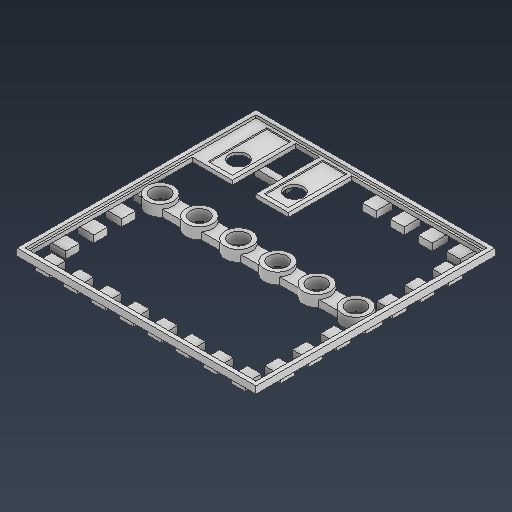
# Autodesk Inventor part: Faceplate
Saved by Autodesk Inventor 2025.3 (Build 293356000, 356)
## iProperties
Created: 2025-09-08
Part Number: Faceplate
Material: Generic
Document SubType Name: Modeling
Designer: tolga
Density: 1 g/cm^3
Appearance: Default
Author: tolga
Autodesk Inventor part; units mm, degrees
ref_plane "YZ Plane" through (0, 0, 0) normal (1, 0, 0) x (0, 1, 0)
ref_plane "XZ Plane" through (0, 0, 0) normal (0, 1, 0) x (-1, 0, 0)
ref_plane "XY Plane" through (0, 0, 0) normal (0, 0, 1) x (1, 0, 0)
sketch "Sketch1" plane through (0, 0, 0) normal (0, 1, 0) x (-1, 0, 0)
  line L0 (0, 0) -> (-171, 0)
  line L1 (-171, 0) -> (-171, -171)
  line L2 (-171, -171) -> (0, -171)
  line L3 (0, -171) -> (0, 0)
  dimension "d0" = 171
  dimension "d1" = 171
  constraints: 8 end point, 2 parallel, 1 horizontal, 1 perpendicular
  measures "d0" distance of L2.end L1.end
  measures "d1" distance of L1.end L0.end
extrude "Extrusion1" add sketch "Sketch1" along normal blind 3
sketch "Sketch3" plane through (0, 3, 0) normal (0, 1, 0) x (1, 0, 0)
  line L0 (4, 64) -> (82, 64) construction
  line L1 (82, 64) -> (82, 4) construction
  line L2 (82, 4) -> (4, 4) construction
  line L3 (4, 4) -> (4, 64) construction
  line L4 (89, 107) -> (167, 107) construction
  line L5 (167, 107) -> (167, 167) construction
  line L6 (167, 167) -> (89, 167) construction
  line L7 (89, 167) -> (89, 107) construction
  line L8 (4, 167) -> (79, 167) construction
  line L9 (79, 167) -> (79, 102) construction
  line L10 (4, 72) -> (4, 167) construction
  line L11 (4, 72) -> (167, 72) construction
  line L12 (167, 72) -> (167, 102) construction
  line L13 (167, 102) -> (79, 102) construction
  line L14 (87, 67) -> (167, 67) construction
  line L15 (167, 67) -> (167, 37) construction
  line L16 (167, 37) -> (87, 37) construction
  line L17 (87, 37) -> (87, 67) construction
  line L18 (87, 32) -> (167, 32) construction
  line L19 (167, 32) -> (167, 7) construction
  line L20 (167, 7) -> (87, 7) construction
  line L21 (87, 7) -> (87, 32) construction
  line L22 (10.3, 32) -> (25.7, 32)
  line L23 (25.7, 32) -> (25.7, 16.6)
  line L24 (25.7, 16.6) -> (10.3, 16.6)
  line L25 (10.3, 16.6) -> (10.3, 32)
  line L26 (10.3, 60) -> (25.7, 60)
  line L27 (10.3, 44.6) -> (10.3, 60)
  line L28 (25.7, 44.6) -> (10.3, 44.6)
  line L29 (25.7, 60) -> (25.7, 44.6)
  line L30 (35.3, 32) -> (50.7, 32)
  line L31 (35.3, 16.6) -> (35.3, 32)
  line L32 (50.7, 16.6) -> (35.3, 16.6)
  line L33 (50.7, 32) -> (50.7, 16.6)
  line L34 (35.3, 60) -> (50.7, 60)
  line L35 (35.3, 44.6) -> (35.3, 60)
  line L36 (50.7, 44.6) -> (35.3, 44.6)
  line L37 (50.7, 60) -> (50.7, 44.6)
  line L38 (60.3, 32) -> (75.7, 32)
  line L39 (60.3, 16.6) -> (60.3, 32)
  line L40 (75.7, 16.6) -> (60.3, 16.6)
  line L41 (75.7, 32) -> (75.7, 16.6)
  line L42 (60.3, 60) -> (75.7, 60)
  line L43 (60.3, 44.6) -> (60.3, 60)
  line L44 (75.7, 44.6) -> (60.3, 44.6)
  line L45 (75.7, 60) -> (75.7, 44.6)
  line L46 (10.3, 60) -> (10.3, 16.6) construction
  line L47 (10.3, 60) -> (75.7, 60) construction
  line L48 (95.3, 135) -> (110.7, 135)
  line L49 (110.7, 135) -> (110.7, 119.6)
  line L50 (110.7, 119.6) -> (95.3, 119.6)
  line L51 (95.3, 119.6) -> (95.3, 135)
  line L52 (95.3, 163) -> (110.7, 163)
  line L53 (95.3, 147.6) -> (95.3, 163)
  line L54 (110.7, 147.6) -> (95.3, 147.6)
  line L55 (110.7, 163) -> (110.7, 147.6)
  line L56 (120.3, 135) -> (135.7, 135)
  line L57 (120.3, 119.6) -> (120.3, 135)
  line L58 (135.7, 119.6) -> (120.3, 119.6)
  line L59 (135.7, 135) -> (135.7, 119.6)
  line L60 (120.3, 163) -> (135.7, 163)
  line L61 (120.3, 147.6) -> (120.3, 163)
  line L62 (135.7, 147.6) -> (120.3, 147.6)
  line L63 (135.7, 163) -> (135.7, 147.6)
  line L64 (145.3, 135) -> (160.7, 135)
  line L65 (145.3, 119.6) -> (145.3, 135)
  line L66 (160.7, 119.6) -> (145.3, 119.6)
  line L67 (160.7, 135) -> (160.7, 119.6)
  line L68 (145.3, 163) -> (160.7, 163)
  line L69 (145.3, 147.6) -> (145.3, 163)
  line L70 (160.7, 147.6) -> (145.3, 147.6)
  line L71 (160.7, 163) -> (160.7, 147.6)
  line L72 (95.3, 163) -> (95.3, 119.6) construction
  line L73 (95.3, 163) -> (160.7, 163) construction
  circle A0 centre (107, 52) radius 12.5 construction
  circle A1 centre (147, 52) radius 12.5 construction
  circle A2 centre (107, 52) radius 4
  circle A3 centre (147, 52) radius 4
  circle A4 centre (99, 19.5) radius 8.1 construction
  circle A5 centre (127, 19.5) radius 8.1 construction
  circle A6 centre (155, 19.5) radius 8.1 construction
  circle A7 centre (99, 19.5) radius 6.4
  circle A8 centre (127, 19.5) radius 6.4
  circle A9 centre (155, 19.5) radius 6.4
  circle A10 centre (155.5, 87) radius 6.5
  circle A11 centre (127.5, 87) radius 6.5
  circle A12 centre (99.5, 87) radius 6.5
  circle A13 centre (71.5, 87) radius 6.5
  circle A14 centre (43.5, 87) radius 6.5
  circle A15 centre (15.5, 87) radius 6.5
  circle A16 centre (61.5, 137) radius 6.5
  circle A17 centre (21.5, 137) radius 6.5
  line L74 (0, 171) -> (0, 0) projected
  line L75 (171, 171) -> (0, 171) projected
  line L76 (171, 0) -> (171, 171) projected
  line L77 (0, 0) -> (171, 0) projected
  point P0 (4, 34)
  point P1 (43, 60)
  point P2 (43, 64)
  point P3 (18, 44.6)
  point P4 (25.7, 52.3)
  point P5 (128, 163)
  point P6 (103, 147.6)
  point P7 (110.7, 155.3)
  point P8 (128, 163)
  point P9 (128, 107)
  point P10 (87, 52)
  point P11 (167, 19.5)
  point P12 (167, 87)
  point P13 (79, 134.5)
  dimension "d9" = 60
  dimension "d10" = 78
  dimension "d11" = 78
  dimension "d12" = 60
  dimension "d17" = 75
  dimension "d20" = 5
  dimension "d21" = 30
  dimension "d22" = 5
  dimension "d23" = 5
  dimension "d27" = 5
  dimension "d28" = 5
  dimension "d31" = 25
  dimension "d32" = 15.4
  dimension "d33" = 15.4
  dimension "d37" = 28
  dimension "d40" = 25
  dimension "d43" = 12.6
  dimension "d44" = 6.3
  dimension "d45" = 4
  dimension "d46" = 14
  dimension "d47" = 11.7
  dimension "d52" = 15.4
  dimension "d53" = 15.4
  dimension "d54" = 28
  dimension "d55" = 25
  dimension "d56" = 12.6
  dimension "d57" = 30
  dimension "d58" = 80
  dimension "d59" = 25
  dimension "d60" = 25
  dimension "d61" = 20
  dimension "d62" = 40
  dimension "d63" = 8
  dimension "d64" = 8
  dimension "d67" = 80
  dimension "d68" = 16.2
  dimension "d69" = 16.2
  dimension "d70" = 16.2
  dimension "d71" = 28
  dimension "d72" = 28
  dimension "d73" = 12
  dimension "d74" = 12.8
  dimension "d75" = 12.8
  dimension "d76" = 12.8
  dimension "d77" = 13
  dimension "d80" = 28
  dimension "d85" = 11.5
  dimension "d86" = 163
  dimension "d87" = 65
  dimension "d88" = 95
  dimension "d89" = 88
  dimension "d90" = 13
  dimension "d91" = 13
  dimension "d92" = 30
  dimension "d93" = 40
  dimension "d94" = 17.5
  dimension "d105" = 4
  dimension "d106" = 4
  dimension "d107" = 4
  dimension "d108" = 4
  dimension "d109" = 4
  dimension "d110" = 4
  dimension "d111" = 7
  dimension "d112" = 4
  constraints: 148 end point, 18 centre point, 14 midpoint, 13 parallel, 11 horizontal, 11 perpendicular, 7 horizontal alignment, 6 collinear, 5 coincident, 2 vertical, 2 vertical alignment, 86 other
  measures "d9" distance between parallel lines of L2 L0
  measures "d10" distance between parallel lines of L3 L1
  measures "d11" distance of L6.end L5.end
  measures "d12" distance of L5.end L4.end
  measures "d17" distance between parallel lines of L10 L9
  measures "d20" distance between parallel lines of L4 L13
  measures "d21" distance between parallel lines of L13 L11
  measures "d22" distance between parallel lines of L11 L14
  measures "d23" distance between parallel lines of L1 L17
  measures "d27" distance between parallel lines of L1 L21
  measures "d28" distance between parallel lines of L16 L18
  measures "d31" distance between parallel lines of L20 L18
  measures "d32" distance of L23.end L24.end
  measures "d33" distance of L22.end L23.end
  measures "d37" distance of L23.end L28.start
  measures "d40" distance of L23.end L32.start
  measures "d43" distance between parallel lines of L2 L24
  measures "d44" distance between parallel lines of L3 L27
  measures "d45" distance between parallel lines of L0 L47
  measures "d46" distance from line of L3 point (18, 44.6)
  measures "d47" distance from line of L0 point (25.7, 52.3)
  measures "d52" distance of L49.end L72.end
  measures "d53" distance of L49.start L49.end
  measures "d54" distance of L49.end L54.start
  measures "d55" distance of L49.end L58.start
  measures "d56" distance between parallel lines of L4 L50
  measures "d57" distance between parallel lines of L14 L16
  measures "d58" distance between parallel lines of L15 L17
  measures "d59" diameter of A0
  measures "d60" diameter of A1
  measures "d61" distance from line of L17 A0.centre
  measures "d62" distance of A0.centre A1.centre
  measures "d63" diameter of A2
  measures "d64" diameter of A3
  measures "d67" distance between parallel lines of L19 L21
  measures "d68" diameter of A4
  measures "d69" diameter of A5
  measures "d70" diameter of A6
  measures "d71" distance of A5.centre A4.centre
  measures "d72" distance of A6.centre A5.centre
  measures "d73" distance from line of L21 A4.centre
  measures "d74" diameter of A7
  measures "d75" diameter of A8
  measures "d76" diameter of A9
  measures "d77" diameter of A10
  measures "d80" distance of A10.centre A11.centre
  measures "d85" distance from line of L12 A10.centre
  measures "d86" distance of L10.start L11.end
  measures "d87" distance of L8.end L9.end
  measures "d88" distance of L10.start L8.start
  measures "d89" distance of L12.end L9.end
  measures "d90" diameter of A16
  measures "d91" diameter of A17
  measures "d92" distance from line of L8 A17.centre
  measures "d93" distance of A17.centre A16.centre
  measures "d94" horizontal distance of point (79, 134.5) A16.centre
  measures "d105" distance between parallel lines of L74 L10
  measures "d106" distance between parallel lines of L75 L8
  measures "d107" distance between parallel lines of L75 L6
  measures "d108" distance between parallel lines of L76 L5
  measures "d109" distance between parallel lines of L76 L12
  measures "d110" distance between parallel lines of L76 L15
  measures "d111" distance between parallel lines of L77 L20
  measures "d112" distance between parallel lines of L76 L19
extrude "Extrusion3" cut sketch "Sketch3" against normal up to surface (3 mm away) contours L22 L23 L24 L25 | L26 L29 L28 L27 | L30 L33 L32 L31 | L34 L37 L36 L35 | L38 L41 L40 L39 | L42 L45 L44 L43 | L48 L49 L50 L51 | L52 L55 L54 L53 | L56 L59 L58 L57 | L60 L63 L62 L61 | L64 L67 L66 L65 | L68 L71 L70 L69 | A2 | A3 | A7 | A8 | A9 | A10 | A11 | A12 | A13 | A14 | A15 | A16 | A17
sketch "Sketch5" plane through (0, 3, 0) normal (0, 1, 0) x (1, 0, 0)
  circle A0 centre (21.5, 137) radius 6.5 construction
  circle A1 centre (61.5, 137) radius 6.5 construction
  line L0 (12.9, 165.8) -> (30.1, 165.8)
  line L1 (30.1, 165.8) -> (30.1, 124)
  line L2 (30.1, 124) -> (12.9, 124)
  line L3 (12.9, 124) -> (12.9, 165.8)
  line L4 (70.1, 124) -> (52.9, 124)
  line L5 (52.9, 124) -> (52.9, 165.8)
  line L6 (52.9, 165.8) -> (70.1, 165.8)
  line L7 (70.1, 165.8) -> (70.1, 124)
  point P0 (0, 0)
  point P1 (21.5, 165.8)
  point P2 (61.5, 165.8)
  point P3 (61.5, 124)
  point P4 (21.5, 124)
  dimension "d99" = 13
  dimension "d100" = 28.8
  dimension "d101" = 17.2
  dimension "d102" = 17.2
  constraints: 16 end point, 4 midpoint, 4 parallel, 2 horizontal, 2 horizontal alignment, 2 perpendicular, 2 vertical alignment
  measures "d99" distance from line of L2 A0.centre
  measures "d100" distance of point (21.5, 165.8) A0.centre
  measures "d101" distance between parallel lines of L1 L3
  measures "d102" distance between parallel lines of L7 L5
extrude "Extrusion5" cut sketch "Sketch5" against normal blind 1
sketch "Sketch7" plane through (0, 3, 0) normal (0, 1, 0) x (1, 0, 0)
  line L0 (52.9, 124) -> (52.9, 165.8) projected
  line L1 (52.9, 165.8) -> (70.1, 165.8) projected
  line L2 (70.1, 165.8) -> (70.1, 124) projected
  line L3 (70.1, 124) -> (52.9, 124) projected
  line L4 (30.1, 165.8) -> (30.1, 124) projected
  line L5 (30.1, 124) -> (12.9, 124) projected
  line L6 (12.9, 124) -> (12.9, 165.8) projected
  line L7 (12.9, 165.8) -> (30.1, 165.8) projected
  circle A0 centre (15.5, 87) radius 6.5 projected
  circle A1 centre (71.5, 87) radius 6.5 projected
  circle A2 centre (99, 19.5) radius 6.4 projected
  line L8 (35.3, 44.6) -> (35.3, 60) projected
  line L9 (35.3, 60) -> (50.7, 60) projected
  line L10 (50.7, 60) -> (50.7, 44.6) projected
  line L11 (50.7, 44.6) -> (35.3, 44.6) projected
  line L12 (50.7, 16.6) -> (35.3, 16.6) projected
  line L13 (35.3, 16.6) -> (35.3, 32) projected
  line L14 (35.3, 32) -> (50.7, 32) projected
  line L15 (50.7, 32) -> (50.7, 16.6) projected
  line L16 (120.3, 119.6) -> (120.3, 135) projected
  line L17 (120.3, 135) -> (135.7, 135) projected
  line L18 (135.7, 135) -> (135.7, 119.6) projected
  line L19 (135.7, 119.6) -> (120.3, 119.6) projected
  circle A3 centre (107, 52) radius 4 projected
  line L20 (145.3, 163) -> (160.7, 163) projected
  line L21 (160.7, 163) -> (160.7, 147.6) projected
  line L22 (160.7, 147.6) -> (145.3, 147.6) projected
  line L23 (145.3, 147.6) -> (145.3, 163) projected
  line L24 (110.7, 135) -> (110.7, 119.6) projected
  line L25 (110.7, 119.6) -> (95.3, 119.6) projected
  line L26 (95.3, 119.6) -> (95.3, 135) projected
  line L27 (95.3, 135) -> (110.7, 135) projected
  line L28 (60.3, 44.6) -> (60.3, 60) projected
  line L29 (60.3, 60) -> (75.7, 60) projected
  line L30 (75.7, 60) -> (75.7, 44.6) projected
  line L31 (75.7, 44.6) -> (60.3, 44.6) projected
  circle A4 centre (127, 19.5) radius 6.4 projected
  circle A5 centre (99.5, 87) radius 6.5 projected
  circle A6 centre (43.5, 87) radius 6.5 projected
  circle A7 centre (155.5, 87) radius 6.5 projected
  line L32 (10.3, 44.6) -> (10.3, 60) projected
  line L33 (10.3, 60) -> (25.7, 60) projected
  line L34 (25.7, 60) -> (25.7, 44.6) projected
  line L35 (25.7, 44.6) -> (10.3, 44.6) projected
  line L36 (25.7, 16.6) -> (10.3, 16.6) projected
  line L37 (10.3, 16.6) -> (10.3, 32) projected
  line L38 (10.3, 32) -> (25.7, 32) projected
  line L39 (25.7, 32) -> (25.7, 16.6) projected
  line L40 (120.3, 147.6) -> (120.3, 163) projected
  line L41 (120.3, 163) -> (135.7, 163) projected
  line L42 (135.7, 163) -> (135.7, 147.6) projected
  line L43 (135.7, 147.6) -> (120.3, 147.6) projected
  circle A8 centre (147, 52) radius 4 projected
  line L44 (145.3, 135) -> (160.7, 135) projected
  line L45 (160.7, 135) -> (160.7, 119.6) projected
  line L46 (160.7, 119.6) -> (145.3, 119.6) projected
  line L47 (145.3, 119.6) -> (145.3, 135) projected
  line L48 (110.7, 147.6) -> (95.3, 147.6) projected
  line L49 (95.3, 147.6) -> (95.3, 163) projected
  line L50 (95.3, 163) -> (110.7, 163) projected
  line L51 (110.7, 163) -> (110.7, 147.6) projected
  line L52 (60.3, 16.6) -> (60.3, 32) projected
  line L53 (60.3, 32) -> (75.7, 32) projected
  line L54 (75.7, 32) -> (75.7, 16.6) projected
  line L55 (75.7, 16.6) -> (60.3, 16.6) projected
  circle A9 centre (155, 19.5) radius 6.4 projected
  circle A10 centre (127.5, 87) radius 6.5 projected
  line L56 (171, 0) -> (171, 171) projected
  line L57 (171, 171) -> (0, 171) projected
  line L58 (0, 171) -> (0, 0) projected
  line L59 (0, 0) -> (171, 0) projected
  line L60 (4.5, 93) -> (166.5, 93)
  line L61 (4.5, 166.5) -> (166.5, 166.5)
  line L62 (166.5, 166.5) -> (166.5, 4.5)
  line L63 (166.5, 4.5) -> (4.5, 4.5)
  line L64 (4.5, 4.5) -> (4.5, 166.5)
  line L65 (30.1, 144.5) -> (52.9, 144.5)
  line L66 (52.9, 139.5) -> (30.1, 139.5)
  line L67 (4.5, 81) -> (166.5, 81)
  line L68 (12.9, 165.8) -> (12.9, 166.5)
  line L69 (30.1, 165.8) -> (30.1, 166.5)
  line L70 (52.9, 124) -> (52.9, 165.8) projected
  line L71 (52.9, 165.8) -> (52.9, 166.5)
  line L72 (70.1, 165.8) -> (70.1, 166.5)
  circle A11 centre (15.5, 87) radius 9.5
  circle A12 centre (43.5, 87) radius 9.5
  circle A13 centre (71.5, 87) radius 9.5
  circle A14 centre (99.5, 87) radius 9.5
  circle A15 centre (127.5, 87) radius 9.5
  circle A16 centre (155.5, 87) radius 9.5
  line L73 (9.9, 168.8) -> (9.9, 121)
  line L74 (9.9, 121) -> (33.1, 121)
  line L75 (33.1, 121) -> (33.1, 168.8)
  line L76 (33.1, 168.8) -> (9.9, 168.8)
  line L77 (49.9, 168.8) -> (73.1, 168.8)
  line L78 (73.1, 168.8) -> (73.1, 121)
  line L79 (73.1, 121) -> (49.9, 121)
  line L80 (49.9, 121) -> (49.9, 168.8)
  line L81 (9.9, 121) -> (4.5, 121)
  point P0 (158, 81)
  point P1 (153, 81)
  point P2 (130, 81)
  point P3 (125, 81)
  point P4 (102, 81)
  point P5 (97, 81)
  point P6 (74, 81)
  point P7 (69, 81)
  point P8 (46, 81)
  point P9 (41, 81)
  point P10 (18, 81)
  point P11 (13, 81)
  point P12 (13, 93)
  point P13 (18, 93)
  point P14 (41, 93)
  point P15 (46, 93)
  point P16 (69, 93)
  point P17 (74, 93)
  point P18 (97, 93)
  point P19 (102, 93)
  point P20 (125, 93)
  point P21 (130, 93)
  point P22 (153, 93)
  point P23 (158, 93)
  point P24 (162.8655, 81)
  point P25 (148.1345, 81)
  point P26 (134.8655, 81)
  point P27 (120.1345, 81)
  point P28 (106.8655, 81)
  point P29 (92.1345, 81)
  point P30 (78.8655, 81)
  point P31 (64.1345, 81)
  point P32 (50.8655, 81)
  point P33 (36.1345, 81)
  point P34 (22.8655, 81)
  point P35 (8.1345, 81)
  point P36 (9.9, 166.5)
  point P37 (8.1345, 93)
  point P38 (22.8655, 93)
  point P39 (36.1345, 93)
  point P40 (50.8655, 93)
  point P41 (64.1345, 93)
  point P42 (78.8655, 93)
  point P43 (92.1345, 93)
  point P44 (106.8655, 93)
  point P45 (120.1345, 93)
  point P46 (134.8655, 93)
  point P47 (148.1345, 93)
  point P48 (162.8655, 93)
  point P49 (73.1, 166.5)
  point P50 (49.9, 139.5)
  point P51 (33.1, 139.5)
  point P52 (49.9, 144.5)
  point P53 (49.9, 166.5)
  point P54 (33.1, 166.5)
  point P55 (33.1, 144.5)
  dimension "d118" = 12
  dimension "d115" = 4.5
  dimension "d116" = 5
  dimension "d117" = 22
  dimension "d119" = 6
  dimension "d122" = 3
  dimension "d125" = 28
  dimension "d130" = 3
  dimension "d131" = 3
  dimension "d132" = 3
  dimension "d133" = 3
  dimension "d134" = 3
  constraints: 38 end point, 13 point on line, 7 perpendicular, 6 centre point, 3 horizontal, 2 parallel, 2 vertical, 22 other
  measures "d115" distance between parallel lines of L57 L61
  measures "d116" distance between parallel lines of L65 L66
  measures "d117" distance between parallel lines of L61 L65
  measures "d122" radial gap between concentric circles of A0 A11
  measures "d125" distance of A0.centre A12.centre
  measures "d130" distance between parallel lines of L6 L73
  measures "d131" distance between parallel lines of L70 L80
  measures "d132" distance between parallel lines of L1 L77
  measures "d133" distance between parallel lines of L2 L78
  measures "d134" distance between parallel lines of L3 L79
extrude "Extrusion6" cut sketch "Sketch7" against normal blind 10 contours L80 L79 L78 L61 L62 L60 A16 A15 A14 A13 A12 A11 L64 L81 L74 L75 L66 | L66 L75 L65 L80 | L65 L75 L61 L80 | L62 L67 A16 L60 | L60 A11 L67 L64 | L62 L63 L64 L67 A11 A12 A13 A14 A15 A16 | A16 L67 A15 L60 | L60 A12 L67 A11 | L60 A10 | A15 L67 A14 L60 | L60 A13 L67 A12 | A10 L67 | A14 L67 A13 L60
sketch "Sketch8" plane through (0, 0, 0) normal (0, -1, 0) x (1, 0, 0)
  line L0 (166.5, -4.5) -> (4.5, -4.5) projected
  line L1 (10.5, 0) -> (20.5, 0)
  line L2 (20.5, 0) -> (20.5, -4.5)
  line L3 (20.5, -4.5) -> (10.5, -4.5)
  line L4 (10.5, -4.5) -> (10.5, 0)
  line L5 (4.5, -121) -> (4.5, -4.5) projected
  line L6 (0, 0) -> (171, 0) projected
  circle A0 centre (155.5, -87) radius 9.5 projected
  circle A1 centre (127.5, -87) radius 9.5 projected
  circle A2 centre (99.5, -87) radius 9.5 projected
  circle A3 centre (71.5, -87) radius 9.5 projected
  circle A4 centre (43.5, -87) radius 9.5 projected
  circle A5 centre (15.5, -87) radius 9.5 projected
  line L7 (4.5, -121) -> (4.5, -4.5) projected
  line L8 (4.5, -4.5) -> (166.5, -4.5) projected
  line L9 (166.5, -4.5) -> (166.5, -166.5) projected
  line L10 (166.5, -166.5) -> (73.1, -166.5) projected
  line L11 (73.1, -166.5) -> (73.1, -121) projected
  line L12 (73.1, -121) -> (49.9, -121) projected
  line L13 (49.9, -121) -> (49.9, -166.5) projected
  line L14 (33.1, -166.5) -> (33.1, -121) projected
  line L15 (33.1, -121) -> (4.5, -121) projected
  line L16 (49.9, -166.5) -> (33.1, -166.5) projected
  circle A6 centre (15.5, -87) radius 6.5 projected
  circle A7 centre (61.5, -137) radius 6.5 projected
  circle A8 centre (71.5, -87) radius 6.5 projected
  circle A9 centre (99.5, -87) radius 6.5 projected
  circle A10 centre (21.5, -137) radius 6.5 projected
  circle A11 centre (43.5, -87) radius 6.5 projected
  circle A12 centre (155.5, -87) radius 6.5 projected
  circle A13 centre (127.5, -87) radius 6.5 projected
  line L17 (171, 0) -> (171, -171) projected
  line L18 (0, 0) -> (171, 0) projected
  line L19 (0, -171) -> (0, 0) projected
  line L20 (171, -171) -> (0, -171) projected
  line L21 (30.5, -4.5) -> (30.5, 0)
  line L22 (40.5, -4.5) -> (30.5, -4.5)
  line L23 (30.5, 0) -> (40.5, 0)
  line L24 (40.5, 0) -> (40.5, -4.5)
  line L25 (50.5, -4.5) -> (50.5, 0)
  line L26 (60.5, -4.5) -> (50.5, -4.5)
  line L27 (50.5, 0) -> (60.5, 0)
  line L28 (60.5, 0) -> (60.5, -4.5)
  line L29 (70.5, -4.5) -> (70.5, 0)
  line L30 (80.5, -4.5) -> (70.5, -4.5)
  line L31 (70.5, 0) -> (80.5, 0)
  line L32 (80.5, 0) -> (80.5, -4.5)
  line L33 (90.5, -4.5) -> (90.5, 0)
  line L34 (100.5, -4.5) -> (90.5, -4.5)
  line L35 (90.5, 0) -> (100.5, 0)
  line L36 (100.5, 0) -> (100.5, -4.5)
  line L37 (110.5, -4.5) -> (110.5, 0)
  line L38 (120.5, -4.5) -> (110.5, -4.5)
  line L39 (110.5, 0) -> (120.5, 0)
  line L40 (120.5, 0) -> (120.5, -4.5)
  line L41 (130.5, -4.5) -> (130.5, 0)
  line L42 (140.5, -4.5) -> (130.5, -4.5)
  line L43 (130.5, 0) -> (140.5, 0)
  line L44 (140.5, 0) -> (140.5, -4.5)
  line L45 (150.5, -4.5) -> (150.5, 0)
  line L46 (160.5, -4.5) -> (150.5, -4.5)
  line L47 (150.5, 0) -> (160.5, 0)
  line L48 (160.5, 0) -> (160.5, -4.5)
  line L49 (160.5, -166.5) -> (150.5, -166.5)
  line L50 (150.5, -166.5) -> (150.5, -171)
  line L51 (150.5, -171) -> (160.5, -171)
  line L52 (160.5, -171) -> (160.5, -166.5)
  line L53 (130.5, -166.5) -> (130.5, -171)
  line L54 (140.5, -166.5) -> (130.5, -166.5)
  line L55 (140.5, -171) -> (140.5, -166.5)
  line L56 (130.5, -171) -> (140.5, -171)
  line L57 (110.5, -166.5) -> (110.5, -171)
  line L58 (120.5, -166.5) -> (110.5, -166.5)
  line L59 (120.5, -171) -> (120.5, -166.5)
  line L60 (110.5, -171) -> (120.5, -171)
  line L61 (90.5, -166.5) -> (90.5, -171)
  line L62 (100.5, -166.5) -> (90.5, -166.5)
  line L63 (100.5, -171) -> (100.5, -166.5)
  line L64 (90.5, -171) -> (100.5, -171)
  line L65 (171, 0) -> (171, -171) projected
  line L66 (166.5, -150.5) -> (171, -150.5)
  line L67 (171, -150.5) -> (171, -140.5)
  line L68 (171, -140.5) -> (166.5, -140.5)
  line L69 (166.5, -140.5) -> (166.5, -150.5)
  line L70 (4.5, -20.5) -> (0, -20.5)
  line L71 (0, -20.5) -> (0, -30.5)
  line L72 (0, -30.5) -> (4.5, -30.5)
  line L73 (4.5, -30.5) -> (4.5, -20.5)
  line L74 (0, -50.5) -> (4.5, -50.5)
  line L75 (4.5, -50.5) -> (4.5, -40.5)
  line L76 (0, -40.5) -> (0, -50.5)
  line L77 (4.5, -40.5) -> (0, -40.5)
  line L78 (0, -70.5) -> (4.5, -70.5)
  line L79 (4.5, -70.5) -> (4.5, -60.5)
  line L80 (0, -60.5) -> (0, -70.5)
  line L81 (4.5, -60.5) -> (0, -60.5)
  line L82 (171, -120.5) -> (166.5, -120.5)
  line L83 (166.5, -120.5) -> (166.5, -130.5)
  line L84 (166.5, -130.5) -> (171, -130.5)
  line L85 (171, -130.5) -> (171, -120.5)
  line L86 (171, -100.5) -> (166.5, -100.5)
  line L87 (166.5, -100.5) -> (166.5, -110.5)
  line L88 (166.5, -110.5) -> (171, -110.5)
  line L89 (171, -110.5) -> (171, -100.5)
  line L90 (171, -80.5) -> (166.5, -80.5)
  line L91 (166.5, -80.5) -> (166.5, -90.5)
  line L92 (166.5, -90.5) -> (171, -90.5)
  line L93 (171, -90.5) -> (171, -80.5)
  line L94 (171, -60.5) -> (166.5, -60.5)
  line L95 (166.5, -60.5) -> (166.5, -70.5)
  line L96 (166.5, -70.5) -> (171, -70.5)
  line L97 (171, -70.5) -> (171, -60.5)
  line L98 (171, -40.5) -> (166.5, -40.5)
  line L99 (166.5, -40.5) -> (166.5, -50.5)
  line L100 (166.5, -50.5) -> (171, -50.5)
  line L101 (171, -50.5) -> (171, -40.5)
  line L102 (171, -20.5) -> (166.5, -20.5)
  line L103 (166.5, -20.5) -> (166.5, -30.5)
  line L104 (166.5, -30.5) -> (171, -30.5)
  line L105 (171, -30.5) -> (171, -20.5)
  point P0 (15.5, 0)
  point P1 (35.5, 0)
  point P2 (55.5, 0)
  point P3 (75.5, 0)
  point P4 (95.5, 0)
  point P5 (115.5, 0)
  point P6 (135.5, 0)
  point P7 (155.5, 0)
  point P8 (155.5, -166.5)
  point P9 (155.5, -171)
  point P10 (135.5, -166.5)
  point P11 (135.5, -171)
  point P12 (115.5, -166.5)
  point P13 (115.5, -171)
  point P14 (95.5, -166.5)
  point P15 (95.5, -171)
  point P16 (4.5, -25.5)
  point P17 (4.5, -30.5)
  point P18 (4.5, -20.5)
  point P19 (0, -20.5)
  point P20 (10.5, -4.5)
  point P21 (40.5, -4.5)
  point P22 (40.5, 0)
  point P23 (30.5, 0)
  point P24 (30.5, -4.5)
  point P25 (60.5, -4.5)
  point P26 (60.5, 0)
  point P27 (50.5, 0)
  point P28 (50.5, -4.5)
  point P29 (80.5, -4.5)
  point P30 (80.5, 0)
  point P31 (70.5, 0)
  point P32 (70.5, -4.5)
  point P33 (100.5, -4.5)
  point P34 (100.5, 0)
  point P35 (90.5, 0)
  point P36 (90.5, -4.5)
  point P37 (120.5, -4.5)
  point P38 (120.5, 0)
  point P39 (110.5, 0)
  point P40 (110.5, -4.5)
  point P41 (140.5, -4.5)
  point P42 (140.5, 0)
  point P43 (130.5, 0)
  point P44 (130.5, -4.5)
  point P45 (160.5, -4.5)
  point P46 (160.5, 0)
  point P47 (150.5, 0)
  point P48 (150.5, -4.5)
  point P49 (110.5, -166.5)
  point P50 (100.5, -166.5)
  point P51 (90.5, -166.5)
  point P52 (4.5, -45.5)
  point P53 (4.5, -65.5)
  point P54 (4.5, -60.5)
  point P55 (0, -60.5)
  point P56 (4.5, -70.5)
  point P57 (0, -40.5)
  point P58 (0, -50.5)
  point P59 (4.5, -50.5)
  dimension "d135" = 10
  dimension "d136" = 6
  dimension "d139" = 20
  dimension "d145" = 10
  dimension "d148" = 20
  dimension "d153" = 16
  dimension "d154" = 10
  dimension "d162" = 10
  dimension "d163" = 16
  dimension "d168" = 20
  dimension "d217" = 6
  dimension "d220" = 20
  constraints: 176 end point, 8 parallel, 7 point on line, 6 horizontal, 4 midpoint, 4 perpendicular, 2 vertical, 159 other
  measures "d135" distance between parallel lines of L4 L2
  measures "d136" distance between parallel lines of L5 L4
  measures "d139" distance of L3.end L21.start
  measures "d145" distance of L50.end L51.end
  measures "d148" distance of L49.end L53.start
  measures "d153" distance between parallel lines of L10 L66
  measures "d154" distance between parallel lines of L66 L68
  measures "d162" distance between parallel lines of L70 L72
  measures "d163" distance between parallel lines of L0 L70
  measures "d168" distance of L71.end L74.start
  measures "d217" distance between parallel lines of L9 L52
  measures "d220" distance of L68.end L82.end
extrude "Extrusion7" add sketch "Sketch8" along normal blind 5 contours L0 L45 L6 L48 | L102 L17 L104 L9 | L0 L41 L6 L44 | L98 L17 L100 L9 | L0 L37 L6 L40 | L94 L17 L96 L9 | L0 L33 L6 L36 | L0 L29 L6 L32 | L86 L17 L88 L9 | L0 L25 L6 L28 | L82 L17 L84 L9 | L0 L21 L6 L24 | L68 L17 L66 L9 | L0 L4 L1 L2 | L52 L20 L50 L10 | L5 L72 L19 L70 | L55 L20 L53 L10 | L5 L74 L19 L77 | L59 L20 L57 L10 | L5 L78 L19 L81 | L63 L20 L61 L10
sketch "Sketch9" plane through (0, -5, 0) normal (0, -1, 0) x (1, 0, 0)
  line L0 (10.5, -4.5) -> (20.5, -4.5) projected
  line L1 (20.5, -4.5) -> (20.5, 0) projected
  line L2 (20.5, 0) -> (10.5, 0) projected
  line L3 (10.5, 0) -> (10.5, -4.5) projected
  line L4 (40.5, 0) -> (30.5, 0) projected
  line L5 (30.5, 0) -> (30.5, -4.5) projected
  line L6 (30.5, -4.5) -> (40.5, -4.5) projected
  line L7 (40.5, -4.5) -> (40.5, 0) projected
  line L8 (60.5, 0) -> (50.5, 0) projected
  line L9 (50.5, 0) -> (50.5, -4.5) projected
  line L10 (50.5, -4.5) -> (60.5, -4.5) projected
  line L11 (60.5, -4.5) -> (60.5, 0) projected
  line L12 (80.5, 0) -> (70.5, 0) projected
  line L13 (70.5, 0) -> (70.5, -4.5) projected
  line L14 (70.5, -4.5) -> (80.5, -4.5) projected
  line L15 (80.5, -4.5) -> (80.5, 0) projected
  line L16 (100.5, 0) -> (90.5, 0) projected
  line L17 (90.5, 0) -> (90.5, -4.5) projected
  line L18 (90.5, -4.5) -> (100.5, -4.5) projected
  line L19 (100.5, -4.5) -> (100.5, 0) projected
  line L20 (120.5, 0) -> (110.5, 0) projected
  line L21 (110.5, 0) -> (110.5, -4.5) projected
  line L22 (110.5, -4.5) -> (120.5, -4.5) projected
  line L23 (120.5, -4.5) -> (120.5, 0) projected
  line L24 (140.5, 0) -> (130.5, 0) projected
  line L25 (130.5, 0) -> (130.5, -4.5) projected
  line L26 (130.5, -4.5) -> (140.5, -4.5) projected
  line L27 (140.5, -4.5) -> (140.5, 0) projected
  line L28 (160.5, 0) -> (150.5, 0) projected
  line L29 (150.5, 0) -> (150.5, -4.5) projected
  line L30 (150.5, -4.5) -> (160.5, -4.5) projected
  line L31 (160.5, -4.5) -> (160.5, 0) projected
  line L32 (52.9, -139.5) -> (30.1, -139.5) projected
  line L33 (30.1, -144.5) -> (52.9, -144.5) projected
  circle A0 centre (15.5, -87) radius 9.5 projected
  circle A1 centre (43.5, -87) radius 9.5 projected
  circle A2 centre (71.5, -87) radius 9.5 projected
  circle A3 centre (99.5, -87) radius 9.5 projected
  circle A4 centre (127.5, -87) radius 9.5 projected
  circle A5 centre (127.5, -87) radius 6.5 projected
  circle A6 centre (99.5, -87) radius 6.5 projected
  circle A7 centre (71.5, -87) radius 6.5 projected
  circle A8 centre (43.5, -87) radius 6.5 projected
  circle A9 centre (15.5, -87) radius 6.5 projected
  line L34 (33.1, -121) -> (33.1, -166.5) projected
  line L35 (49.9, -166.5) -> (49.9, -121) projected
  line L36 (10.5, -4.5) -> (20.5, -4.5)
  line L37 (20.5, -4.5) -> (20.5, -14.5)
  line L38 (20.5, -14.5) -> (10.5, -14.5)
  line L39 (10.5, -14.5) -> (10.5, -4.5)
  line L40 (40.5, -14.5) -> (30.5, -14.5)
  line L41 (30.5, -14.5) -> (30.5, -4.5)
  line L42 (40.5, -4.5) -> (40.5, -14.5)
  line L43 (30.5, -4.5) -> (40.5, -4.5)
  line L44 (60.5, -14.5) -> (50.5, -14.5)
  line L45 (50.5, -14.5) -> (50.5, -4.5)
  line L46 (60.5, -4.5) -> (60.5, -14.5)
  line L47 (50.5, -4.5) -> (60.5, -4.5)
  line L48 (80.5, -14.5) -> (70.5, -14.5)
  line L49 (70.5, -14.5) -> (70.5, -4.5)
  line L50 (80.5, -4.5) -> (80.5, -14.5)
  line L51 (70.5, -4.5) -> (80.5, -4.5)
  line L52 (100.5, -14.5) -> (90.5, -14.5)
  line L53 (90.5, -14.5) -> (90.5, -4.5)
  line L54 (100.5, -4.5) -> (100.5, -14.5)
  line L55 (90.5, -4.5) -> (100.5, -4.5)
  line L56 (120.5, -14.5) -> (110.5, -14.5)
  line L57 (110.5, -14.5) -> (110.5, -4.5)
  line L58 (120.5, -4.5) -> (120.5, -14.5)
  line L59 (110.5, -4.5) -> (120.5, -4.5)
  line L60 (140.5, -14.5) -> (130.5, -14.5)
  line L61 (130.5, -14.5) -> (130.5, -4.5)
  line L62 (140.5, -4.5) -> (140.5, -14.5)
  line L63 (130.5, -4.5) -> (140.5, -4.5)
  line L64 (160.5, -14.5) -> (150.5, -14.5)
  line L65 (150.5, -14.5) -> (150.5, -4.5)
  line L66 (160.5, -4.5) -> (160.5, -14.5)
  line L67 (150.5, -4.5) -> (160.5, -4.5)
  line L68 (30.1, -139.5) -> (30.1, -144.5)
  line L69 (52.9, -139.5) -> (52.9, -144.5)
  line L70 (0, -171) -> (0, -70.5) projected
  line L71 (166.5, -140.5) -> (166.5, -150.5) projected
  line L72 (166.5, -150.5) -> (171, -150.5) projected
  line L73 (171, -150.5) -> (171, -140.5) projected
  line L74 (171, -140.5) -> (166.5, -140.5) projected
  line L75 (171, -130.5) -> (171, -120.5) projected
  line L76 (171, -120.5) -> (166.5, -120.5) projected
  line L77 (166.5, -120.5) -> (166.5, -130.5) projected
  line L78 (166.5, -130.5) -> (171, -130.5) projected
  line L79 (171, -110.5) -> (171, -100.5) projected
  line L80 (171, -100.5) -> (166.5, -100.5) projected
  line L81 (166.5, -100.5) -> (166.5, -110.5) projected
  line L82 (166.5, -110.5) -> (171, -110.5) projected
  line L83 (171, -70.5) -> (171, -60.5) projected
  line L84 (171, -60.5) -> (166.5, -60.5) projected
  line L85 (166.5, -60.5) -> (166.5, -70.5) projected
  line L86 (166.5, -70.5) -> (171, -70.5) projected
  line L87 (171, -50.5) -> (171, -40.5) projected
  line L88 (171, -40.5) -> (166.5, -40.5) projected
  line L89 (166.5, -40.5) -> (166.5, -50.5) projected
  line L90 (166.5, -50.5) -> (171, -50.5) projected
  line L91 (171, -30.5) -> (171, -20.5) projected
  line L92 (171, -20.5) -> (166.5, -20.5) projected
  line L93 (166.5, -20.5) -> (166.5, -30.5) projected
  line L94 (166.5, -30.5) -> (171, -30.5) projected
  line L95 (4.5, -93) -> (166.5, -93) projected
  line L96 (4.5, -81) -> (166.5, -81) projected
  circle A10 centre (155.5, -87) radius 6.5 projected
  circle A11 centre (155.5, -87) radius 9.5 projected
  line L97 (171, -70.5) -> (166.5, -70.5) projected
  line L98 (166.5, -70.5) -> (166.5, -100.5) projected
  line L99 (166.5, -100.5) -> (171, -100.5) projected
  line L100 (171, -70.5) -> (171, -100.5) projected
  line L101 (4.5, -70.5) -> (0, -70.5) projected
  line L102 (0, -171) -> (0, -70.5) projected
  line L103 (90.5, -171) -> (0, -171) projected
  line L104 (90.5, -171) -> (90.5, -166.5) projected
  line L105 (90.5, -166.5) -> (73.1, -166.5) projected
  line L106 (73.1, -166.5) -> (73.1, -121) projected
  line L107 (73.1, -121) -> (49.9, -121) projected
  line L108 (49.9, -121) -> (49.9, -166.5) projected
  line L109 (49.9, -166.5) -> (33.1, -166.5) projected
  line L110 (33.1, -166.5) -> (33.1, -121) projected
  line L111 (33.1, -121) -> (4.5, -121) projected
  line L112 (4.5, -121) -> (4.5, -70.5) projected
  circle A12 centre (61.5, -137) radius 6.5 projected
  circle A13 centre (21.5, -137) radius 6.5 projected
  line L113 (160.5, -166.5) -> (150.5, -166.5) projected
  line L114 (150.5, -166.5) -> (150.5, -171) projected
  line L115 (150.5, -171) -> (160.5, -171) projected
  line L116 (160.5, -171) -> (160.5, -166.5) projected
  line L117 (140.5, -166.5) -> (130.5, -166.5) projected
  line L118 (130.5, -166.5) -> (130.5, -171) projected
  line L119 (130.5, -171) -> (140.5, -171) projected
  line L120 (140.5, -171) -> (140.5, -166.5) projected
  line L121 (120.5, -166.5) -> (110.5, -166.5) projected
  line L122 (110.5, -166.5) -> (110.5, -171) projected
  line L123 (110.5, -171) -> (120.5, -171) projected
  line L124 (120.5, -171) -> (120.5, -166.5) projected
  line L125 (100.5, -166.5) -> (90.5, -166.5) projected
  line L126 (90.5, -166.5) -> (90.5, -171) projected
  line L127 (90.5, -171) -> (100.5, -171) projected
  line L128 (100.5, -171) -> (100.5, -166.5) projected
  line L129 (0, -60.5) -> (0, -70.5) projected
  line L130 (0, -70.5) -> (4.5, -70.5) projected
  line L131 (4.5, -70.5) -> (4.5, -60.5) projected
  line L132 (4.5, -60.5) -> (0, -60.5) projected
  line L133 (0, -40.5) -> (0, -50.5) projected
  line L134 (0, -50.5) -> (4.5, -50.5) projected
  line L135 (4.5, -50.5) -> (4.5, -40.5) projected
  line L136 (4.5, -40.5) -> (0, -40.5) projected
  line L137 (4.5, -30.5) -> (4.5, -20.5) projected
  line L138 (4.5, -20.5) -> (0, -20.5) projected
  line L139 (0, -20.5) -> (0, -30.5) projected
  line L140 (0, -30.5) -> (4.5, -30.5) projected
  line L141 (160.5, -166.5) -> (150.5, -166.5)
  line L142 (150.5, -166.5) -> (150.5, -156.5)
  line L143 (150.5, -156.5) -> (160.5, -156.5)
  line L144 (160.5, -156.5) -> (160.5, -166.5)
  line L145 (166.5, -150.5) -> (156.5, -150.5)
  line L146 (156.5, -150.5) -> (156.5, -140.5)
  line L147 (156.5, -140.5) -> (166.5, -140.5)
  line L148 (166.5, -140.5) -> (166.5, -150.5)
  line L149 (166.5, -20.5) -> (156.5, -20.5)
  line L150 (156.5, -20.5) -> (156.5, -30.5)
  line L151 (156.5, -30.5) -> (166.5, -30.5)
  line L152 (166.5, -30.5) -> (166.5, -20.5)
  line L153 (4.5, -70.5) -> (14.5, -70.5)
  line L154 (14.5, -70.5) -> (14.5, -60.5)
  line L155 (14.5, -60.5) -> (4.5, -60.5)
  line L156 (4.5, -60.5) -> (4.5, -70.5)
  line L157 (166.5, -130.5) -> (156.5, -130.5)
  line L158 (156.5, -120.5) -> (166.5, -120.5)
  line L159 (166.5, -120.5) -> (166.5, -130.5)
  line L160 (156.5, -130.5) -> (156.5, -120.5)
  line L161 (166.5, -110.5) -> (156.5, -110.5)
  line L162 (156.5, -100.5) -> (166.5, -100.5)
  line L163 (166.5, -100.5) -> (166.5, -110.5)
  line L164 (156.5, -110.5) -> (156.5, -100.5)
  line L165 (140.5, -166.5) -> (130.5, -166.5)
  line L166 (130.5, -156.5) -> (140.5, -156.5)
  line L167 (140.5, -156.5) -> (140.5, -166.5)
  line L168 (130.5, -166.5) -> (130.5, -156.5)
  line L169 (120.5, -166.5) -> (110.5, -166.5)
  line L170 (110.5, -156.5) -> (120.5, -156.5)
  line L171 (120.5, -156.5) -> (120.5, -166.5)
  line L172 (110.5, -166.5) -> (110.5, -156.5)
  line L173 (100.5, -166.5) -> (90.5, -166.5)
  line L174 (90.5, -156.5) -> (100.5, -156.5)
  line L175 (100.5, -156.5) -> (100.5, -166.5)
  line L176 (90.5, -166.5) -> (90.5, -156.5)
  line L177 (166.5, -40.5) -> (156.5, -40.5)
  line L178 (156.5, -40.5) -> (156.5, -50.5)
  line L179 (156.5, -50.5) -> (166.5, -50.5)
  line L180 (166.5, -50.5) -> (166.5, -40.5)
  line L181 (166.5, -60.5) -> (156.5, -60.5)
  line L182 (156.5, -60.5) -> (156.5, -70.5)
  line L183 (156.5, -70.5) -> (166.5, -70.5)
  line L184 (166.5, -70.5) -> (166.5, -60.5)
  line L185 (14.5, -40.5) -> (4.5, -40.5)
  line L186 (4.5, -40.5) -> (4.5, -50.5)
  line L187 (14.5, -50.5) -> (14.5, -40.5)
  line L188 (4.5, -50.5) -> (14.5, -50.5)
  line L189 (14.5, -20.5) -> (4.5, -20.5)
  line L190 (4.5, -20.5) -> (4.5, -30.5)
  line L191 (14.5, -30.5) -> (14.5, -20.5)
  line L192 (4.5, -30.5) -> (14.5, -30.5)
  line L193 (4.5, -93) -> (0, -93)
  line L194 (4.5, -81) -> (0, -81)
  line L195 (166.5, -93) -> (171, -93)
  line L196 (166.5, -81) -> (171, -81)
  point P0 (0, 0)
  point P1 (135.5, -30.5)
  point P2 (135.5, -30.5)
  point P3 (49.9, -144.5)
  point P4 (49.9, -139.5)
  point P5 (33.1, -139.5)
  point P6 (33.1, -144.5)
  point P7 (150.5, -4.5)
  point P8 (40.5, -4.5)
  point P9 (22.8655, -81)
  point P10 (22.8655, -93)
  point P11 (36.1345, -93)
  point P12 (36.1345, -81)
  point P13 (8.1345, -81)
  point P14 (8.1345, -93)
  point P15 (120.1345, -93)
  point P16 (120.1345, -81)
  point P17 (106.8655, -81)
  point P18 (106.8655, -93)
  point P19 (134.8655, -93)
  point P20 (134.8655, -81)
  point P21 (92.1345, -93)
  point P22 (92.1345, -81)
  point P23 (78.8655, -81)
  point P24 (78.8655, -93)
  point P25 (64.1345, -93)
  point P26 (64.1345, -81)
  point P27 (50.8655, -81)
  point P28 (50.8655, -93)
  point P29 (4.5, -40.5)
  point P30 (4.5, -20.5)
  point P31 (148.1345, -81)
  point P32 (148.1345, -93)
  point P33 (162.8655, -93)
  point P34 (162.8655, -81)
  point P35 (0, -81)
  point P36 (0, -93)
  dimension "d181" = 10
  dimension "d184" = 20
  dimension "d225" = 10
  dimension "d226" = 10
  dimension "d227" = 10
  dimension "d228" = 10
  dimension "d229" = 10
  dimension "d230" = 10
  dimension "d231" = 10
  dimension "d232" = 10
  dimension "d235" = 20
  dimension "d242" = 20
  dimension "d249" = 20
  dimension "d256" = 20
  constraints: 180 end point, 11 parallel, 7 horizontal, 7 perpendicular, 7 point on line, 3 vertical, 1 coincident, 141 other
  measures "d181" distance of L0.end L37.end
  measures "d184" distance of L38.end L40.end
  measures "d225" distance of L142.end L143.end
  measures "d226" distance of L141.end L142.end
  measures "d227" distance of L146.end L147.end
  measures "d228" distance of L145.end L146.end
  measures "d229" distance of L151.end L150.end
  measures "d230" distance of L150.end L149.end
  measures "d231" distance of L155.end L154.end
  measures "d232" distance of L154.end L153.end
  measures "d235" distance of L71.start point (166.5, -120.5)
  measures "d242" distance of L142.end L166.start
  measures "d249" distance of L149.end L177.end
  measures "d256" distance of L101.start point (4.5, -50.5)
extrude "Extrusion8" add sketch "Sketch9" against normal up to surface (5 mm away) contours L0 L37 L38 L39 | L42 L40 L41 L6 | L46 L44 L45 L10 | L50 L48 L49 L14 | L54 L52 L53 L18 | L58 L56 L57 L22 | L62 L60 L61 L26 | L66 L64 L65 L30 | L69 L33 L35 L32 | L35 L33 L34 L32 | L34 L33 L68 L32 | L112 L96 A0 L95 | L193 L70 L194 L112 | L176 L174 L175 L125 | L95 A9 A0 | A0 L96 A9 L95 | A0 L96 A9 | L95 A9 L96 A0 | A0 L96 A1 L95 | L131 L155 L154 L153 | L95 A8 A1 | A1 L96 A8 L95 | A1 L96 A8 | L95 A8 L96 A1 | A1 L96 A2 L95 | L95 A7 A2 | A2 L96 A7 L95 | A2 L96 A7 | L95 A7 L96 A2 | A2 L96 A3 L95 | L95 A6 A3 | A3 L96 A6 L95 | A3 L96 A6 | L95 A6 L96 A3 | A3 L96 A4 L95 | L95 A5 A4 | A4 L96 A5 L95 | A4 L96 A5 | L95 A5 L96 A4 | A4 L96 A11 L95 | A11 L96 A10 L95 | L95 A10 A11 | A11 L96 A10 | A11 L96 L98 L95 | L95 A10 L96 A11 | L98 L196 L100 L195 | L81 L161 L164 L162 | L183 L182 L181 L85 | L71 L145 L146 L147 | L157 L160 L158 L77 | L179 L178 L177 L89 | L151 L150 L149 L93 | L113 L142 L143 L144 | L117 L168 L166 L167 | L121 L172 L170 L171 | L185 L187 L188 L135 | L137 L189 L191 L192
sketch "Sketch10" plane through (0, -5, 0) normal (0, -1, 0) x (1, 0, 0)
  line L0 (171, -171) -> (0, -171) projected
  line L1 (0, -171) -> (0, 0) projected
  line L2 (0, 0) -> (171, 0) projected
  line L3 (171, 0) -> (171, -171) projected
  line L4 (2.7, -2.7) -> (2.7, -168.3)
  line L5 (2.7, -168.3) -> (168.3, -168.3)
  line L6 (168.3, -168.3) -> (168.3, -2.7)
  line L7 (168.3, -2.7) -> (2.7, -2.7)
  dimension "d261" = 2.7
  constraints: 8 end point, 3 other
  measures "d261" distance between parallel lines of L1 L4
extrude "Extrusion9" cut sketch "Sketch10" against normal up to surface (5 mm away)
fillet "Fillet1" radius 1 23 edges at (2.7, 0, -65.5) (2.7, 0, -87) (2.7, 0, -45.5) (2.7, 0, -25.5) (15.5, 0, -2.7) (35.5, 0, -2.7) (55.5, 0, -2.7) (75.5, 0, -2.7) (95.5, 0, -2.7) (115.5, 0, -2.7) (135.5, 0, -2.7) (155.5, 0, -2.7) (95.5, 0, -168.3) (115.5, 0, -168.3) (135.5, 0, -168.3) (155.5, 0, -168.3) (168.3, 0, -145.5) (168.3, 0, -125.5) (168.3, 0, -105.5) (168.3, 0, -65.5) (168.3, 0, -45.5) (168.3, 0, -25.5) (168.3, 0, -87)
sketch "Sketch11" plane through (0, 3, 0) normal (0, 1, 0) x (1, 0, 0)
  line L0 (171, 0) -> (171, 171) projected
  line L1 (171, 171) -> (0, 171) projected
  line L2 (0, 171) -> (0, 0) projected
  line L3 (0, 0) -> (171, 0) projected
  line L4 (3, 168) -> (168, 168)
  line L5 (168, 168) -> (168, 3)
  line L6 (168, 3) -> (3, 3)
  line L7 (3, 3) -> (3, 168)
  dimension "d265" = 3
  constraints: 8 end point, 3 other
  measures "d265" distance between parallel lines of L1 L4
extrude "Extrusion10" add sketch "Sketch11" along normal blind 2
equation "\"d11\" = d10"
equation "\"d12\" = d9"
equation "\"d43\" = d37 - d33"
equation "\"d56\" = d43"
equation "\"d60\" = d59"
equation "\"d61\" = -0.5 * d62 + 0.5 * d58"
equation "\"d64\" = d63"
equation "\"d69\" = d68"
equation "\"d70\" = d68"
equation "\"d72\" = d71"
equation "\"d73\" = -d71 + 0.5 * d67"
equation "\"d75\" = d74"
equation "\"d76\" = d74"
body "Solid1"
